bike_light_part (Autodesk Fusion 360 design; units mm, degrees)
Autodesk Fusion 360 part; units mm, degrees
note: some values were not read from the file. Set by a fixed rule: which sketch regions a step uses.
sketch "Sketch1" plane through (0, 0, 0) normal (0, 1, 0) x (1, 0, 0)
  line L0 (0, 0) -> (-15, 0)
  line L1 (-15, 0) -> (-15, -15)
  line L2 (-15, -15) -> (0, -15)
  line L3 (0, -15) -> (0, 0)
  line L4 (-15, 0) -> (-40, -20.9775)
  line L5 (-40, -20.9775) -> (-40, -35.9775)
  line L6 (-40, -35.9775) -> (-25, -35.9775)
  line L7 (-25, -35.9775) -> (0, -15)
  line L8 (0, -15) -> (-15, 0)
  line L9 (-15, -15) -> (0, 0)
  circle A0 centre (-7.5, -7.5) radius 3.5
  dimension "d1" = 15
  dimension "d2" = 15
  dimension "d3" = 15
  dimension "d4" = 40
  dimension "d5" = 15
  dimension "d6" = 25
  dimension "d19" = 7
  constraint horizontal L0
  constraint vertical L1
  constraint horizontal L2
  constraint vertical L3
  constraint coincident L0.start L3.end
  constraint parallel L1 L5
  constraint perpendicular L5 L6
  constraint midpoint L9 A0.centre
  measures "d1" distance of L0.start L0.end
  measures "d2" distance of L0.start L2.end
  measures "d3" distance of L5.end L6.end
  measures "d4" angle of L2 L7
  measures "d5" distance of L4.end L5.end
  measures "d6" distance of L1 L5
  measures "d19" diameter of A0
extrude "Extrude1" add sketch "Sketch1" along normal blind 12
sketch "Sketch2" plane through (0, 0, 35.9775) normal (0, 0, 1) x (-1, 0, 0)
  line L0 (40, 0) -> (25, 0)
  line L1 (25, 0) -> (25, -12)
  line L2 (25, -12) -> (40, -12)
  line L3 (40, -12) -> (40, 0)
  line L4 (25, 0) -> (40, -12)
  line L5 (40, 0) -> (25, -12)
  circle A0 centre (32.5, -6) radius 2.5
  circle A1 centre (32.5, -6) radius 4.5
  dimension "d9" = 5
  dimension "d10" = 9
  constraint coincident L0.end L1.start
  constraint coincident L2.end L3.start
  constraint coincident L0.start L3.end
  constraint coincident L1.end L2.start
  constraint midpoint L5 A0.centre
  constraint concentric A0 A1
  measures "d9" diameter of A0
  measures "d10" diameter of A1
extrude "Extrude2" cut sketch "Sketch2" against normal blind 36 contours L4 L5 A0 | L4 L5 A0 | L4 L5 A0 | L4 L5 A0
extrude "Extrude3" cut sketch "Sketch2" against normal blind 18 from surface at -12.5 contours L4 L5 A0 A1 | L4 L5 A0 A1 | L4 L5 A0 A1 | L4 L5 A0 A1
chamfer "Chamfer1" distance 2 angle 45 1 edges at (-30.1692, 5.096, 23.4775)
chamfer "Chamfer2" distance 2 distance2 12 1 edges at (-40, 6, 35.9775) measured on face at (-40, 8, 30.9775)
extrude "Extrude4" cut sketch "Sketch1" along normal blind 21 contours L8 L9 A0 | L8 L9 A0 | L8 L9 A0 | L8 L9 A0
fillet "Fillet1" radius 3 6 edges at (-15, 6, 0) (0, 6, 0) (0, 6, 15) (-40, 6, 20.9775) (-40, 6, 33.9775) (-25, 6, 35.9775)
equation "d2 = d1"
